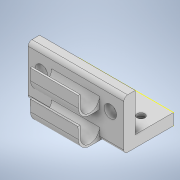
# Autodesk Inventor part: giá đỡ vòi
Saved by Autodesk Inventor 2020 (Build 240168000, 168)
## iProperties
Created: 2022-09-22
Part Number: giá đỡ vòi
Material: Generic
Document SubType Name: Modeling
Designer: ASUS
Density: 1 g/cm^3
Appearance: Default
Author: ASUS
Autodesk Inventor part; units mm, degrees
ref_plane "YZ Plane" through (0, 0, 0) normal (1, 0, 0) x (0, 1, 0)
ref_plane "XZ Plane" through (0, 0, 0) normal (0, 1, 0) x (-1, 0, 0)
ref_plane "XY Plane" through (0, 0, 0) normal (0, 0, 1) x (1, 0, 0)
sketch "Sketch1" plane through (0, 0, 0) normal (0, 0, 1) x (1, 0, 0)
  line L0 (0, 0) -> (25, 0)
  line L1 (25, 0) -> (25, 26)
  line L2 (25, 26) -> (0, 26)
  line L3 (0, 26) -> (0, 0)
  dimension "d0" = 25
  dimension "d1" = 26
  constraints: 8 end point, 2 parallel, 1 horizontal, 1 perpendicular
  measures "d0" distance of L2.end L1.end
  measures "d1" distance of L1.end L0.end
extrude "Extrusion1" add sketch "Sketch1" along normal blind 6
sketch "Sketch2" plane through (0, 0, 0) normal (0, 0, -1) x (-1, 0, 0)
  line L0 (0, 26) -> (0, 0) projected
  line L1 (-25, 0) -> (-25, 26) projected
  line L2 (0, 0) -> (-25, 0)
  line L3 (-25, 0) -> (-25, 6)
  line L4 (-25, 6) -> (0, 6)
  line L5 (0, 6) -> (0, 0)
  point P0 (0, 6)
  dimension "d95" = 6
  constraints: 8 end point, 2 parallel, 1 horizontal, 1 perpendicular, 1 point on line
  measures "d95" distance between parallel lines of L4 L2
extrude "Extrusion2" add sketch "Sketch2" along normal blind 20
move faces "Move1" translate (25, 0, 0) faces at (25, 10.6667, 4)
sketch "Sketch7" plane through (0, 0, 6) normal (0, 0, 1) x (1, 0, 0)
  line L0 (50, 26) -> (0, 26) projected
  line L1 (50, 0) -> (0, 0) projected
  line L2 (12.3464, 26) -> (37.3464, 26)
  line L3 (37.3464, 26) -> (37.3464, 0)
  line L4 (37.3464, 0) -> (12.3464, 0)
  line L5 (12.3464, 0) -> (12.3464, 26)
  point P0 (37.3464, 26)
  dimension "d29" = 25
  constraints: 8 end point, 2 parallel, 2 point on line, 1 horizontal, 1 perpendicular
  measures "d29" distance of L3.end L4.end
extrude "Extrusion7" add sketch "Sketch7" along normal blind 12
ref_plane "Work Plane1" through (37.3464, 0, 5) normal (1, 0, 0) x (0, 0, -1)
sketch "Sketch8" plane through (37.3464, 0, 5) normal (1, 0, 0) x (0, 0, -1)
  line L0 (-1, 26) -> (-13, 26) projected
  line L1 (-1, 12) -> (-1, 20)
  line L2 (-1, 26) -> (-1, 0) projected
  line L3 (-1, 12) -> (-1, 18) projected
  line L4 (-1, 12) -> (-1, 20)
  line L5 (-1, 20) -> (-1, 12)
  line L6 (-1, 26) -> (-1, 0) projected
  line L7 (-13, 26) -> (-13, 0) projected
  line L8 (-1, 26) -> (-13, 26) projected
  arc A0 (-11, 20) -> (-1, 20) centre (-6, 20) ccw
  line L9 (-1, 0) -> (-1, 26) projected
  arc A1 (-11, 20) -> (-6, 15) centre (-6, 20) ccw
  arc A2 (-11, 6) -> (-1, 6) centre (-6, 6) ccw
  line L10 (-1, 0) -> (-13, 0) projected
  line L11 (-11.2095, 12) -> (-12.2923, 12)
  line L12 (-13, 0) -> (-13, 26) projected
  line L13 (-12.0828, 6) -> (-6.0791, 6) construction
  line L14 (-11, 6) -> (-11.2095, 12)
  line L15 (-11, 6) -> (-4.9963, 6) construction
  line L16 (25, 0) -> (-1, 0) projected
  line L17 (-1, 0) -> (-1, 6)
  line L18 (-1, 14) -> (-1, 20)
  line L19 (-1, 0) -> (-1, 26) projected
  line L20 (-11.2095, 26) -> (-11.2095, 26)
  line L21 (-11, 20) -> (-11.2095, 26)
  line L22 (-11, 20) -> (-4.9963, 20) construction
  line L23 (-11, 20) -> (-11.2095, 26)
  line L24 (-11, 20) -> (-4.9963, 20) construction
  line L25 (-12, 20) -> (-12.2095, 26)
  line L26 (-12, 20) -> (-5.9963, 20) construction
  line L27 (-12.2095, 26) -> (-11.2095, 26)
  line L28 (-6, 14) -> (-1, 14)
  arc A3 (-12, 20) -> (-6, 14) centre (-6, 20) ccw
  arc A4 (-1, 15.6834) -> (-1, 24.3166) centre (-6, 20) ccw
  line L29 (-1, 0) -> (-13, 0) projected
  line L30 (-1, 0) -> (-6.0791, 0)
  arc A5 (-12.0791, 6) -> (-6.0791, 0) centre (-6.0791, 6) ccw
  line L31 (-1, 6) -> (-1, 0)
  line L32 (-12.0791, 6) -> (-12.2923, 12)
  point P0 (5, 0)
  point P1 (-10, 12)
  point P2 (-1, 14)
  dimension "d76" = 10
  dimension "d77" = 6
  dimension "d78" = 5
  dimension "d80" = 10
  dimension "d81" = 5
  dimension "d82" = 6
  dimension "d85" = 92
  dimension "d86" = 92
  dimension "d87" = 92
  dimension "d91" = 92
  constraints: 42 end point, 12 point on circle, 7 point on line, 6 centre point, 6 horizontal, 4 equal length, 3 coincident, 2 vertical, 1 collinear, 1 perpendicular, 1 tangent, 9 other
  measures "d76" diameter of A0
  measures "d77" distance from line of L0 A0.centre
  measures "d78" distance from line of L2 A0.centre
  measures "d80" diameter of A2
  measures "d81" distance from line of L2 A2.centre
  measures "d82" distance from line of L10 A2.centre
  measures "d85" angle of L15 L14
  measures "d86" angle of L22 L21
  measures "d87" angle of L24 L23
  measures "d91" angle of L26 L25
extrude "Extrusion15" cut sketch "Sketch8" against normal through all contours L2 A0 L21 L0 | L25 A3 L28 L1 L2 A2 L14 L11 L32 A5 L10 L7 L0
fillet "Fillet3" radius 2 3 edges at (43.6732, 0, 6) (6.1732, 0, 6) (25, 26, 6)
sketch "Sketch11" plane through (0, 0, -20) normal (0, -1, 0) x (1, 0, 0)
  circle A0 centre (7, 10) radius 3
  line L0 (0, 0) -> (0, 24) projected
  line L1 (50, 0) -> (0, 0) projected
  point P0 (0, 20)
  dimension "d96" = 6
  dimension "d97" = 7
  dimension "d98" = 10
  constraints: 1 centre point
  measures "d96" diameter of A0
  measures "d97" distance from line of L0 A0.centre
  measures "d98" distance from line of L1 A0.centre
hole "Hole1" at (7, 0, -10) direction (0, 1, 0) diameter 4 end through all counterbore diameter 6.5 counterbore depth 4.5
sketch "Sketch12" plane through (0, 0, 6) normal (0, 0, 1) x (1, 0, 0)
  circle A0 centre (7, 16) radius 3
  line L0 (50, 26) -> (0, 26) projected
  line L1 (0, 24) -> (0, 2) projected
  point P0 (0, 0)
  dimension "d106" = 6
  dimension "d107" = 10
  dimension "d108" = 7
  constraints: 1 centre point
  measures "d106" diameter of A0
  measures "d107" distance from line of L0 A0.centre
  measures "d108" distance from line of L1 A0.centre
hole "Hole2" at (7, 16, 6) direction (0, 0, -1) diameter 4 end through all counterbore diameter 6.5 counterbore depth 4.5
sketch "Sketch13" plane through (0, 0, -20) normal (0, 0, -1) x (-1, 0, 0)
  line L0 (-50, 6) -> (0, 6) projected
  line L1 (-25, 6) -> (-25, 0)
  line L2 (-50, 0) -> (0, 0) projected
  constraints: 2 end point, 2 midpoint
ref_plane "Work Plane3" through (25, 6, -20) normal (1, 0, 0) x (0, -1, 0)
mirror "Mirror1" about plane through (25, 6, -20) normal (1, 0, 0) of "Hole2", "Hole1"
body "Solid1"
